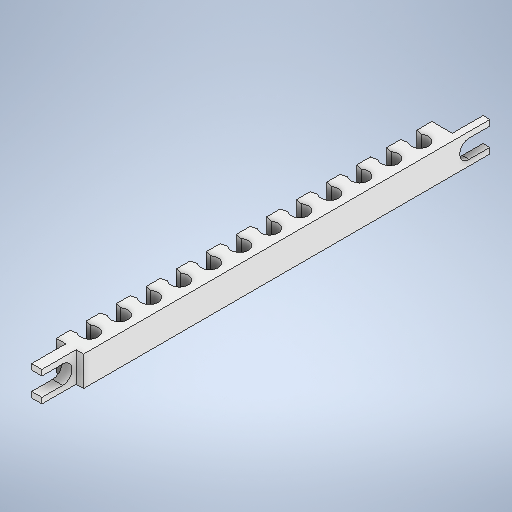
# Autodesk Inventor part: Hose Clamp V4
Saved by Autodesk Inventor 2025 (Build 290162000, 162)
## iProperties
Created: 2023-05-24
Part Number: Hose Clamp V4
Material: ABS Plastic
Document SubType Name: Modeling
Designer: cfangmeier3
Density: 1.06 g/cm^3
Appearance: Smooth - White
Author: cfangmeier3
Autodesk Inventor part; units mm, degrees
ref_plane "YZ Plane" through (0, 0, 0) normal (1, 0, 0) x (0, 1, 0)
ref_plane "XZ Plane" through (0, 0, 0) normal (0, 1, 0) x (-1, 0, 0)
ref_plane "XY Plane" through (0, 0, 0) normal (0, 0, 1) x (1, 0, 0)
sketch "Sketch1" plane through (0, 0, 0) normal (0, 1, 0) x (-1, 0, 0)
  line L0 (0, 69.85) -> (0, -69.85)
  line L1 (2.54, 69.85) -> (10.16, 69.85)
  line L2 (10.16, 67.31) -> (10.16, 64.77)
  line L3 (10.16, 64.77) -> (7.9419, 64.217)
  line L4 (10.16, 58.674) -> (7.9419, 59.227)
  arc A0 (7.9419, 64.217) -> (7.9419, 59.227) centre (5.9783, 61.722) ccw
  line L5 (0, 69.85) -> (2.54, 69.85)
  line L6 (6.604, 69.85) -> (2.794, 69.85)
  line L7 (2.794, 69.85) -> (2.794, 82.55)
  line L8 (2.794, 82.55) -> (6.604, 82.55)
  line L9 (6.604, 82.55) -> (6.604, 69.85)
  line L10 (2.54, -69.85) -> (2.54, -81.28)
  line L11 (2.54, -81.28) -> (0, -81.28)
  line L12 (0, -81.28) -> (0, -69.85)
  line L13 (5.9783, 61.722) -> (7.9419, 61.722) construction
  line L14 (7.9419, 61.722) -> (7.9419, 59.227) construction
  line L15 (7.9419, 61.722) -> (7.9419, 64.217) construction
  line L16 (10.16, 67.31) -> (10.16, 69.85)
  line L17 (10.16, -66.802) -> (10.16, -69.85)
  line L18 (10.16, -69.85) -> (2.54, -69.85)
  line L19 (10.16, 58.674) -> (10.16, 56.134)
  line L20 (10.16, 56.134) -> (10.16, 53.594)
  line L21 (10.16, 53.594) -> (7.9419, 53.041)
  line L22 (7.9419, 50.546) -> (7.9419, 53.041) construction
  arc A1 (7.9419, 53.041) -> (7.9419, 48.051) centre (5.9783, 50.546) ccw
  line L23 (7.9419, 50.546) -> (7.9419, 48.051) construction
  line L24 (10.16, 47.498) -> (7.9419, 48.051)
  line L25 (10.16, 47.498) -> (10.16, 44.958)
  line L26 (5.9783, 50.546) -> (7.9419, 50.546) construction
  line L27 (10.16, 44.958) -> (10.16, 42.418)
  line L28 (10.16, 42.418) -> (7.9419, 41.865)
  line L29 (7.9419, 39.37) -> (7.9419, 41.865) construction
  arc A2 (7.9419, 41.865) -> (7.9419, 36.875) centre (5.9783, 39.37) ccw
  line L30 (7.9419, 39.37) -> (7.9419, 36.875) construction
  line L31 (10.16, 36.322) -> (7.9419, 36.875)
  line L32 (10.16, 36.322) -> (10.16, 33.782)
  line L33 (5.9783, 39.37) -> (7.9419, 39.37) construction
  line L34 (10.16, 33.782) -> (10.16, 31.242)
  line L35 (10.16, 31.242) -> (7.9419, 30.689)
  line L36 (7.9419, 28.194) -> (7.9419, 30.689) construction
  arc A3 (7.9419, 30.689) -> (7.9419, 25.699) centre (5.9783, 28.194) ccw
  line L37 (7.9419, 28.194) -> (7.9419, 25.699) construction
  line L38 (10.16, 25.146) -> (7.9419, 25.699)
  line L39 (10.16, 25.146) -> (10.16, 22.606)
  line L40 (5.9783, 28.194) -> (7.9419, 28.194) construction
  line L41 (10.16, 22.606) -> (10.16, 20.066)
  line L42 (10.16, 20.066) -> (7.9419, 19.513)
  line L43 (7.9419, 17.018) -> (7.9419, 19.513) construction
  arc A4 (7.9419, 19.513) -> (7.9419, 14.523) centre (5.9783, 17.018) ccw
  line L44 (7.9419, 17.018) -> (7.9419, 14.523) construction
  line L45 (10.16, 13.97) -> (7.9419, 14.523)
  line L46 (10.16, 13.97) -> (10.16, 11.43)
  line L47 (5.9783, 17.018) -> (7.9419, 17.018) construction
  line L48 (10.16, 11.43) -> (10.16, 8.89)
  line L49 (10.16, 8.89) -> (7.9419, 8.337)
  line L50 (7.9419, 5.842) -> (7.9419, 8.337) construction
  arc A5 (7.9419, 8.337) -> (7.9419, 3.347) centre (5.9783, 5.842) ccw
  line L51 (7.9419, 5.842) -> (7.9419, 3.347) construction
  line L52 (10.16, 2.794) -> (7.9419, 3.347)
  line L53 (10.16, 2.794) -> (10.16, 0.254)
  line L54 (5.9783, 5.842) -> (7.9419, 5.842) construction
  line L55 (10.16, 0.254) -> (10.16, -2.286)
  line L56 (10.16, -2.286) -> (7.9419, -2.839)
  line L57 (7.9419, -5.334) -> (7.9419, -2.839) construction
  arc A6 (7.9419, -2.839) -> (7.9419, -7.829) centre (5.9783, -5.334) ccw
  line L58 (7.9419, -5.334) -> (7.9419, -7.829) construction
  line L59 (10.16, -8.382) -> (7.9419, -7.829)
  line L60 (10.16, -8.382) -> (10.16, -10.922)
  line L61 (5.9783, -5.334) -> (7.9419, -5.334) construction
  line L62 (10.16, -10.922) -> (10.16, -13.462)
  line L63 (10.16, -13.462) -> (7.9419, -14.015)
  line L64 (7.9419, -16.51) -> (7.9419, -14.015) construction
  arc A7 (7.9419, -14.015) -> (7.9419, -19.005) centre (5.9783, -16.51) ccw
  line L65 (7.9419, -16.51) -> (7.9419, -19.005) construction
  line L66 (10.16, -19.558) -> (7.9419, -19.005)
  line L67 (10.16, -19.558) -> (10.16, -22.098)
  line L68 (5.9783, -16.51) -> (7.9419, -16.51) construction
  line L69 (10.16, -22.098) -> (10.16, -24.638)
  line L70 (10.16, -24.638) -> (7.9419, -25.191)
  line L71 (7.9419, -27.686) -> (7.9419, -25.191) construction
  arc A8 (7.9419, -25.191) -> (7.9419, -30.181) centre (5.9783, -27.686) ccw
  line L72 (7.9419, -27.686) -> (7.9419, -30.181) construction
  line L73 (10.16, -30.734) -> (7.9419, -30.181)
  line L74 (10.16, -30.734) -> (10.16, -33.274)
  line L75 (5.9783, -27.686) -> (7.9419, -27.686) construction
  line L76 (10.16, -33.274) -> (10.16, -35.814)
  line L77 (10.16, -35.814) -> (7.9419, -36.367)
  line L78 (7.9419, -38.862) -> (7.9419, -36.367) construction
  arc A9 (7.9419, -36.367) -> (7.9419, -41.357) centre (5.9783, -38.862) ccw
  line L79 (7.9419, -38.862) -> (7.9419, -41.357) construction
  line L80 (10.16, -41.91) -> (7.9419, -41.357)
  line L81 (10.16, -41.91) -> (10.16, -44.45)
  line L82 (5.9783, -38.862) -> (7.9419, -38.862) construction
  line L83 (10.16, -44.45) -> (10.16, -46.99)
  line L84 (10.16, -46.99) -> (7.9419, -47.543)
  line L85 (7.9419, -50.038) -> (7.9419, -47.543) construction
  arc A10 (7.9419, -47.543) -> (7.9419, -52.533) centre (5.9783, -50.038) ccw
  line L86 (7.9419, -50.038) -> (7.9419, -52.533) construction
  line L87 (10.16, -53.086) -> (7.9419, -52.533)
  line L88 (10.16, -53.086) -> (10.16, -55.626)
  line L89 (5.9783, -50.038) -> (7.9419, -50.038) construction
  line L90 (10.16, -55.626) -> (10.16, -58.166)
  line L91 (10.16, -58.166) -> (7.9419, -58.719)
  line L92 (7.9419, -61.214) -> (7.9419, -58.719) construction
  arc A11 (7.9419, -58.719) -> (7.9419, -63.709) centre (5.9783, -61.214) ccw
  line L93 (7.9419, -61.214) -> (7.9419, -63.709) construction
  line L94 (10.16, -64.262) -> (7.9419, -63.709)
  line L95 (10.16, -64.262) -> (10.16, -66.802)
  line L96 (5.9783, -61.214) -> (7.9419, -61.214) construction
  point P0 (0, 0)
  point P1 (2.794, 69.85)
  dimension "d1" = 7.62
  dimension "d5" = 104
  dimension "d7" = 3.175
  dimension "d8" = 2.286
  dimension "d12" = 2.54
  dimension "d27" = 12.7
  dimension "d28" = 3.81
  dimension "d29" = 2.794
  dimension "d66" = 139.7
  dimension "d67" = 69.85
  dimension "d76" = 10.16
  dimension "d77" = 2.54
  dimension "d87" = 11.43
  dimension "d88" = 2.54
  dimension "d89" = 4.9899
  dimension "d90" = 2.54
  dimension "d91" = 11.176
  dimension "d94" = 11.176
  constraints: 194 end point, 24 point on circle, 12 centre point, 7 vertical, 4 horizontal alignment, 3 horizontal, 3 perpendicular, 3 vertical alignment, 2 equal length, 2 parallel, 1 coincident, 1 midpoint, 1 point on line, 176 other
  measures "d1" distance of L1.start L1.end
  measures "d5" angle of L3 L2
  measures "d7" radius of A0
  measures "d8" distance of L2.end L3.end
  measures "d12" distance of L2.start L2.end
  measures "d27" distance of L8.end L6.start
  measures "d28" distance of L7.end L8.end
  measures "d29" distance of L0.start L6.end
  measures "d66" distance of L0.start L0.end
  measures "d67" distance of L0.start point (0, 0)
  measures "d76" distance of L1.end L0.start
  measures "d77" distance of L2.start L1.end
  measures "d87" distance of L10.start L10.end
  measures "d88" distance of L10.end L11.end
  measures "d89" distance of L3.end L4.end
  measures "d90" distance of L4.start L19.end
  measures "d91" distance of L2.start L19.end
  measures "d94" distance of L2.start L20.start
extrude "Extrusion1" add sketch "Sketch1" along normal blind 11.1125
sketch "Sketch3" plane through (0, 0, 69.85) normal (1, 0, 0) x (0, 0, -1)
  line L0 (158.877, 5.5563) -> (143.383, 5.5562) construction
  line L1 (158.877, 8.9853) -> (143.383, 8.9852)
  line L2 (143.383, 2.1272) -> (158.877, 2.1273)
  arc A0 (158.877, 2.1273) -> (158.877, 8.9853) centre (158.877, 5.5563) ccw
  arc A1 (143.383, 8.9852) -> (143.383, 2.1272) centre (143.383, 5.5562) ccw
  line L3 (151.13, 0) -> (151.13, 11.1125) projected
  line L4 (0, 11.1125) -> (151.13, 11.1125) projected
  line L5 (-20.447, 5.5563) -> (-4.953, 5.5563) construction
  line L6 (-20.447, 2.1273) -> (-4.953, 2.1272)
  line L7 (-4.953, 8.9853) -> (-20.447, 8.9853)
  arc A2 (-20.447, 8.9853) -> (-20.447, 2.1273) centre (-20.447, 5.5563) ccw
  arc A3 (-4.953, 2.1272) -> (-4.953, 8.9853) centre (-4.953, 5.5563) ccw
  line L8 (-12.7, 0) -> (-12.7, 11.1125) projected
  point P0 (69.85, 0)
  point P1 (151.13, 5.5563)
  point P2 (-12.7, 5.5563)
  point P3 (-12.7, 8.9853)
  point P4 (-12.7, 2.1272)
  point P5 (151.13, 2.1272)
  point P6 (151.13, 8.9853)
  dimension "d45" = 11.1125
  dimension "d46" = 5.5563
  dimension "d47" = 7.747
  dimension "d48" = 7.747
  dimension "d49" = 6.858
  dimension "d50" = 6.858
  constraints: 16 end point, 8 point on circle, 8 tangent, 4 centre point, 3 midpoint, 2 horizontal, 2 parallel, 1 collinear, 1 horizontal alignment
  measures "d45" distance of L3.start L3.end
  measures "d46" distance from line of L4 point (151.13, 5.556)
  measures "d47" distance from line of L3 L0.end
  measures "d48" distance from line of L8 L5.end
  measures "d49" distance between parallel lines of L1 L2
  measures "d50" distance between parallel lines of L7 L6
extrude "Extrusion2" cut sketch "Sketch3" against normal through all contours L3 L2 A1 L1 | L8 L7 A3 L6
body "Solid1"
